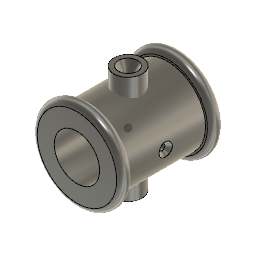
_bearing.7b8933d9-a149-4dbc-b5f2-1142ab0e05e8 (Autodesk Fusion 360 design; units mm, degrees)
Autodesk Fusion 360 part; units mm, degrees
note: some values were not read from the file. Chosen so that the rebuilt part matches the saved one: which bodies a step acts on.
sketch "Sketch1" plane through (0, 0, 0) normal (0, 1, 0) x (1, 0, 0)
  circle A0 centre (0, 0) radius 20
  dimension "d1" = 40
  constraint coincident A0.centre origin
  measures "d1" diameter of A0
extrude "Extrude1" add sketch "Sketch1" along normal blind 21 and the other way blind 21 makes body 1
sketch "Sketch2" plane through (0, -21, 0) normal (0, -1, 0) x (1, 0, 0)
  circle A0 centre (0, 0) radius 20
  circle A1 centre (0, 0) radius 24
  dimension "d6" = 48
  constraint coincident A0.centre A1.centre
  measures "d6" diameter of A1
extrude "Extrude2" add sketch "Sketch2" along normal blind 6 contours A0 | A1 bodies 1
sketch "Sketch3" plane through (0, 21, 0) normal (0, 1, 0) x (-1, 0, 0)
  circle A0 centre (0, 0) radius 20
  circle A1 centre (0, 0) radius 24
  dimension "d9" = 48
  constraint concentric A0 A1
  measures "d9" diameter of A1
extrude "Extrude3" add sketch "Sketch3" along normal blind 6 contours A0 | A1 bodies 1
fillet "Fillet1" radius 3 4 edges at (22.3759, 27, -8.6788) (22.3759, 21, -8.6788) (-22.3759, -21, -8.6788) (-22.3759, -27, -8.6788) on bodies 1
sketch "Sketch4" plane through (0, -27, 0) normal (0, -1, 0) x (1, 0, 0)
  circle A0 centre (0, 0) radius 21
  circle A1 centre (0, 0) radius 12
  dimension "d13" = 24
  constraint coincident A0.centre A1.centre
  measures "d13" diameter of A1
extrude "Extrude4" cut sketch "Sketch4" against normal blind 60 contours A1 bodies 1
sketch "Sketch5" plane through (0, 0, 0) normal (0, 0, 1) x (1, 0, 0)
  circle A0 centre (0, 0) radius 7.5
  dimension "d16" = 15
  constraint coincident A0.centre origin
  measures "d16" diameter of A0
extrude "Extrude5" add sketch "Sketch5" along normal blind 28.5 and the other way blind 28.5 separate body makes body 2
sketch "Sketch6" plane through (0, -27, 0) normal (0, -1, 0) x (1, 0, 0)
  circle A0 centre (0, 0) radius 12
  circle A1 centre (0, 0) radius 21
  circle A2 centre (0, 0) radius 12
  constraint coincident A0.centre A1.centre
extrude "Extrude6" cut sketch "Sketch6" against normal blind 85 contours A0 A2 bodies 2 makes body 3 at (-7.4815, 0.5258, 22.1262)
sketch "Sketch7" plane through (0, 0, 0) normal (1, 0, 0) x (0, 1, 0)
  line L0 (-7.5, -28.5) -> (7.5, -28.5)
  line L1 (8.6822, -28.5) -> (8.6822, -19.5)
  line L2 (8.6822, -19.5) -> (0, -19.5)
  line L3 (0, -19.5) -> (2, -19.5)
  line L4 (2, -19.5) -> (2, -23.3038)
  line L5 (2, -23.3038) -> (5, -28.5)
  line L6 (2, -23.3038) -> (8.3509, -23.3038) construction
  line L7 (5, -28.5) -> (0, -28.5)
  line L8 (0, -28.5) -> (0, -19.5)
  line L9 (2, -19.5) -> (0, -19.5)
  line L10 (0, -28.5) -> (5, -28.5)
  point P0 (0, -28.5)
  dimension "d23" = 9
  dimension "d24" = 2
  dimension "d25" = 60
  dimension "d26" = 5
  constraint perpendicular L0 L1
  constraint perpendicular L1 L2
  constraint parallel L2 L3
  constraint perpendicular L2 L4
  constraint horizontal L6
  constraint coincident L0 L5.end
  constraint coincident P0 L7.end
  constraint perpendicular L3 L8
  constraint parallel L0 L10
  constraint coincident L5.end L7.start
  measures "d23" distance of L1.start L1.end
  measures "d24" distance of L2.end L3.end
  measures "d25" angle of L5 L6
  measures "d26" distance of P0 L5.end
revolve "Revolve1" cut sketch "Sketch7" angle 360 about axis through (0, 0, -28.5) along (0, 0, 1) bodies 1 2
mirror "Mirror1" about plane through (0, 0, 0) normal (0, 0, 1) of "Revolve1"
sketch "Sketch8" plane through (0, 0, 0) normal (1, 0, 0) x (0, 1, 0)
  line L0 (27, 12) -> (27, -12)
  line L1 (0, 28.5) -> (0, 19.5)
  line L2 (0, 19.5) -> (2, 19.5)
  line L3 (0, 28.5) -> (5, 28.5)
  line L4 (5, 28.5) -> (2, 23.3038)
  line L5 (5, 28.5) -> (10.8655, 28.5) construction
  line L6 (2, 19.5) -> (2, 23.3038)
  point P0 (0, 28.5)
  dimension "d29" = 9
  dimension "d30" = 2
  dimension "d31" = 5
  dimension "d32" = 120
  constraint coincident P0 L1.start
  constraint parallel L0 L1
  constraint perpendicular L1 L2
  constraint perpendicular L1 L3
  constraint horizontal L5
  constraint perpendicular L2 L6
  constraint coincident L4.end L6.end
  measures "d29" distance of P0 L1.end
  measures "d30" distance of L1.end L2.end
  measures "d31" distance of P0 L3.end
  measures "d32" angle of L4 L5
revolve "Revolve2" cut sketch "Sketch8" angle 360 about axis through (0, 0, 28.5) along (0, 0, -1) bodies 3
sketch "Sketch9" plane through (0, 0, 0) normal (1, 0, 0) x (0, 1, 0)
  circle A0 centre (0, 0) radius 1.5
  dimension "d34" = 3
  constraint coincident A0.centre origin
  measures "d34" diameter of A0
ref_plane "WorkPlane1" through (20, 0, 0) normal (1, 0, 0) x (0, 1, 0)
sketch "Sketch10" plane through (20, 0, 0) normal (1, 0, 0) x (0, 1, 0)
  circle A0 centre (0, 0) radius 1.5
  dimension "d36" = 3
  constraint coincident A0.centre origin
  measures "d36" diameter of A0
extrude "Extrude7" cut sketch "Sketch10" against normal blind 15 bodies 1
chamfer "Chamfer1" distance 2 angle 45 2 edges at (19.9437, 0, -1.5) (19.9437, 0, 1.5) on bodies 1
